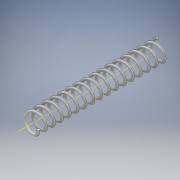
# Autodesk Inventor part: spring-25mm
Saved by Autodesk Inventor 2018 (Build 220112000, 112)
## iProperties
Created: 2017-11-05
Part Number: spring-25mm
Material: Generic
Document SubType Name: Modeling
Designer: Jurjen
Density: 1 g/cm^3
Appearance: Default
Author: Jurjen
Autodesk Inventor part; units mm, degrees
ref_plane "YZ Plane" through (0, 0, 0) normal (1, 0, 0) x (0, 1, 0)
ref_plane "XY Plane" through (0, 0, 0) normal (0, 0, 1) x (1, 0, 0)
sketch "Sketch1" plane through (0, 0, 0) normal (0, 0, 1) x (1, 0, 0)
  circle A0 centre (1.6, 0) radius 0.25
  line L0 (1.6, 0) -> (0, 0)
  line L1 (0, 0) -> (0, 20)
  dimension "d0" = 20
  dimension "d1" = 0.5
  dimension "d2" = 1.6
  constraints: 4 end point, 1 centre point, 1 horizontal, 1 perpendicular
  measures "d0" distance of L0.end L1.end
  measures "d1" diameter of A0
  measures "d2" distance of L0.start L0.end
coil "Coil1" sketch "Sketch1" operation add axis through (0, 0, 0) along (0, 1, 0) pitch 1.5 turns 16.666667 hand right
sketch "Sketch2" plane through (0, 0, 0) normal (0, 1, 0) x (-1, 0, 0)
  line L0 (-1.85, 0) -> (-1.35, 0) projected
  circle A0 centre (0, 0) radius 1.85
  constraints: 1 coincident, 1 horizontal alignment, 2 other
body "Solid1"
